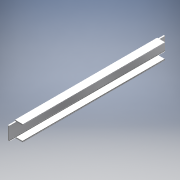
# Autodesk Inventor part: NASA-20-FR-01
Saved by Autodesk Inventor 2019 (Build 230136000, 136)
## iProperties
Created: 2019-09-05
Part Number: NASA-20-FR-01
Material: Aluminum 6061
Description: FRONT PLATE
Document SubType Name: Modeling
Designer: Rick Szalay
Stock Number: 1630T31
Density: 2.7 g/cm^3
Appearance: Aluminum - Flat
Author: Rick Szalay
Autodesk Inventor part; units mm, degrees
ref_plane "YZ Plane" through (0, 0, 0) normal (1, 0, 0) x (0, 1, 0)
ref_plane "XZ Plane" through (0, 0, 0) normal (0, 1, 0) x (-1, 0, 0)
ref_plane "XY Plane" through (0, 0, 0) normal (0, 0, 1) x (1, 0, 0)
sketch "Sketch3" plane through (0, 0, 0) normal (0, 0, 1) x (1, 0, 0)
  line L0 (0, 38.1) -> (0, -38.1)
  line L1 (0, 38.1) -> (38.1, 38.1)
  line L2 (38.1, 38.1) -> (38.1, 33.02)
  line L3 (38.1, 33.02) -> (3.302, 33.02)
  line L4 (3.302, 33.02) -> (3.302, -33.02)
  line L5 (3.302, -33.02) -> (38.1, -33.02)
  line L6 (38.1, -33.02) -> (38.1, -38.1)
  line L7 (38.1, -38.1) -> (0, -38.1)
  line L8 (0, 0) -> (3.302, 0) construction
  dimension "d7" = 76.2
  dimension "d8" = 3.302
  dimension "d9" = 66.04
  dimension "d10" = 38.1
  constraints: 18 end point, 6 perpendicular, 2 horizontal, 2 midpoint, 1 coincident, 1 vertical, 1 other
  measures "d7" distance of L0.start L0.end
  measures "d8" distance between parallel lines of L0 L4
  measures "d9" distance between parallel lines of L5 L3
  measures "d10" distance of L0.start L1.end
extrude "Extrusion3" add sketch "Sketch3" along normal mid plane 501.396
fillet "Fillet1" radius 3.175 4 edges at (38.1, 33.02, 0) (38.1, -33.02, 0) (3.302, -33.02, 0) (3.302, 33.02, 0)
sketch "Sketch4" plane through (0, -38.1, 250.698) normal (-1, 0, 0) x (0, 0, 1)
  line L0 (0, 76.2) -> (-501.396, 76.2) projected
  line L1 (-501.396, 76.2) -> (-466.598, 76.2)
  line L2 (-466.598, 76.2) -> (-466.598, 71.12)
  line L3 (-466.598, 71.12) -> (-501.396, 71.12)
  line L4 (-501.396, 71.12) -> (-501.396, 76.2)
  line L5 (0, 67.945) -> (-501.396, 67.945) projected
  line L6 (-501.396, 8.255) -> (0, 8.255) projected
  line L7 (-501.396, 0) -> (0, 0) projected
  line L8 (-501.396, 0) -> (0, 0) projected
  line L9 (-501.396, 0) -> (-466.598, 0)
  line L10 (-466.598, 0) -> (-466.598, 5.08)
  line L11 (-466.598, 5.08) -> (-501.396, 5.08)
  line L12 (-501.396, 5.08) -> (-501.396, 0)
  line L13 (0, 5.08) -> (-501.396, 5.08) projected
  line L14 (-501.396, 71.12) -> (0, 71.12) projected
  point P0 (-250.698, 38.1)
  dimension "d14" = 34.798
  constraints: 16 end point, 4 parallel, 3 collinear, 2 horizontal, 2 perpendicular
  measures "d14" distance between parallel lines of L4 L2
extrude "Extrusion4" cut sketch "Sketch4" against normal through all
mirror "Mirror1" about plane through (0, 0, 0) normal (0, 0, 1) of "Extrusion4"
fillet "Fillet3" radius 3.175 4 edges at (3.2385, 33.02, -250.698) (3.2385, -33.02, -250.698) (3.2385, 33.02, 250.698) (3.2385, -33.02, 250.698)
equation "\"d11\" = Length"
equation "\"Length\" = 501.396"
body "Solid2"
